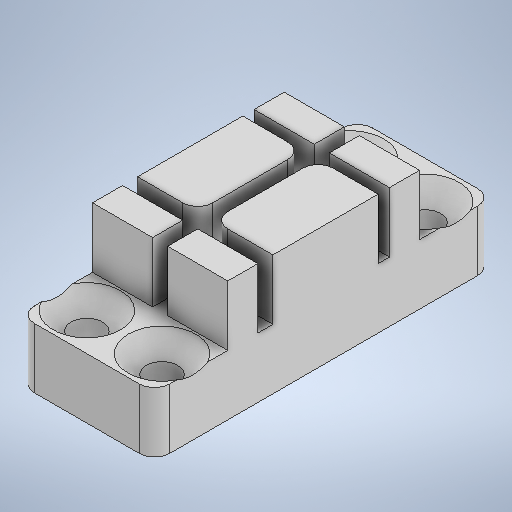
# Autodesk Inventor part: jonction de courroie
Saved by Autodesk Inventor 2025.2 (Build 292293000, 293)
## iProperties
Created: 2025-03-28
Part Number: jonction de courroie
Material: Générique
Document SubType Name: Modeling
Designer: enezl
Density: 1 g/cm^3
Appearance: Par défaut
Author: enezl
Autodesk Inventor part; units mm, degrees
ref_plane "YZ Plane" through (0, 0, 0) normal (1, 0, 0) x (0, 1, 0)
ref_plane "XZ Plane" through (0, 0, 0) normal (0, 1, 0) x (-1, 0, 0)
ref_plane "XY Plane" through (0, 0, 0) normal (0, 0, 1) x (1, 0, 0)
sketch "Esquisse1" plane through (0, 0, 0) normal (0, 1, 0) x (-1, 0, 0)
  line L0 (-7, 22.5) -> (7, 22.5)
  line L1 (9, 20.5) -> (9, -20.5)
  line L2 (7, -22.5) -> (-7, -22.5)
  line L3 (-9, -20.5) -> (-9, 20.5)
  line L4 (-9, 22.5) -> (9, -22.5) construction
  line L5 (9, 22.5) -> (-9, -22.5) construction
  line L6 (-5, -17.5) -> (5, -17.5) construction
  line L7 (5, -17.5) -> (5, 17.5) construction
  line L8 (5, 17.5) -> (-5, 17.5) construction
  line L9 (-5, 17.5) -> (-5, -17.5) construction
  line L10 (-5, -17.5) -> (5, 17.5) construction
  line L11 (5, -17.5) -> (-5, 17.5) construction
  arc A0 (9, 20.5) -> (7, 22.5) centre (7, 20.5) ccw
  arc A1 (-7, 22.5) -> (-9, 20.5) centre (-7, 20.5) ccw
  arc A2 (-9, -20.5) -> (-7, -22.5) centre (-7, -20.5) ccw
  arc A3 (7, -22.5) -> (9, -20.5) centre (7, -20.5) ccw
  point P0 (0, 0)
  dimension "d0" = 18
  dimension "d1" = 45
  dimension "d3" = 4
  dimension "d4" = 5
  dimension "d25" = 2
  constraints: 24 end point, 8 point on circle, 8 point on line, 8 tangent, 4 centre point, 4 coincident, 4 midpoint, 4 parallel, 3 equal radius, 2 horizontal, 2 perpendicular
  measures "d0" distance of L4.end L5.end
  measures "d1" distance of L5.start L4.end
  measures "d3" distance between parallel lines of L1 L7
  measures "d4" distance between parallel lines of L0 L8
  measures "d25" radius of A0
extrude "Extrusion1" add sketch "Esquisse1" against normal blind 8
hole "Perçage1" at (-5, 0, 17.5) at (5, 0, 17.5) at (5, 0, -17.5) at (-5, 0, -17.5) direction (0, -1, 0) diameter 4.2 end through all countersink diameter 9 countersink angle 90
sketch "Esquisse2" plane through (0, 0, 0) normal (0, 1, 0) x (1, 0, 0)
  line L0 (-9, -20.5) -> (-9, 20.5) construction
  line L1 (9, 12.75) -> (-9, 12.75) construction
  line L2 (-9, 12.75) -> (-9, -12.75) construction
  line L3 (-9, -12.75) -> (9, -12.75) construction
  line L4 (9, -12.75) -> (9, 12.75) construction
  line L5 (9, 12.75) -> (-9, -12.75) construction
  line L6 (-9, 12.75) -> (9, -12.75) construction
  line L7 (9, 7.25) -> (3, 7.25)
  line L8 (1, 5.25) -> (1, -4.75)
  line L9 (3, -6.75) -> (9, -6.75)
  line L10 (9, -6.75) -> (9, 7.25)
  arc A0 (1, -4.75) -> (3, -6.75) centre (3, -4.75) ccw
  arc A1 (3, 7.25) -> (1, 5.25) centre (3, 5.25) ccw
  line L11 (9, -12.75) -> (1, -12.75)
  line L12 (1, -12.75) -> (1, -8.75)
  line L13 (1, -8.75) -> (9, -8.75)
  line L14 (9, -8.75) -> (9, -12.75)
  line L15 (9, 12.75) -> (1, 12.75)
  line L16 (1, 12.75) -> (1, 8.75)
  line L17 (1, 8.75) -> (9, 8.75)
  line L18 (9, 8.75) -> (9, 12.75)
  line L19 (0, -22.5) -> (0, 22.5)
  line L20 (-7, -22.5) -> (7, -22.5) construction
  line L21 (7, 22.5) -> (-7, 22.5) construction
  line L22 (-9, -12.75) -> (-9, 12.75) construction
  line L23 (-9, 7.25) -> (-3, 7.25)
  line L24 (-1, 5.25) -> (-1, -4.75)
  line L25 (-3, -6.75) -> (-9, -6.75)
  line L26 (-9, -6.75) -> (-9, 7.25)
  arc A2 (-3, -6.75) -> (-1, -4.75) centre (-3, -4.75) ccw
  arc A3 (-1, 5.25) -> (-3, 7.25) centre (-3, 5.25) ccw
  line L27 (-9, -12.75) -> (-1, -12.75)
  line L28 (-1, -12.75) -> (-1, -8.75)
  line L29 (-1, -8.75) -> (-9, -8.75)
  line L30 (-9, -8.75) -> (-9, -12.75)
  line L31 (-9, 12.75) -> (-1, 12.75)
  line L32 (-1, 12.75) -> (-1, 8.75)
  line L33 (-1, 8.75) -> (-9, 8.75)
  line L34 (-9, 8.75) -> (-9, 12.75)
  point P0 (0, 0)
  point P1 (-9, -22.5)
  point P2 (-9, 22.5)
  dimension "d17" = 2
  dimension "d19" = 14
  dimension "d20" = 4
  dimension "d21" = 2
  dimension "d22" = 4
  dimension "d23" = 1.5
  dimension "d24" = 1
  constraints: 64 end point, 14 symmetric about line, 8 parallel, 8 point on circle, 5 midpoint, 4 centre point, 4 horizontal, 4 perpendicular, 4 tangent, 3 point on line, 2 collinear, 1 equal radius, 1 vertical, 2 other
  measures "d17" distance between parallel lines of L9 L13
  measures "d19" distance of L9.end L7.start
  measures "d20" distance of L11.end L12.end
  measures "d21" radius of A0
  measures "d22" distance of L15.end L16.end
  measures "d23" distance between parallel lines of L7 L17
  measures "d24" distance from line of point (0, 0) L8
extrude "Extrusion2" add sketch "Esquisse2" along normal blind 8
